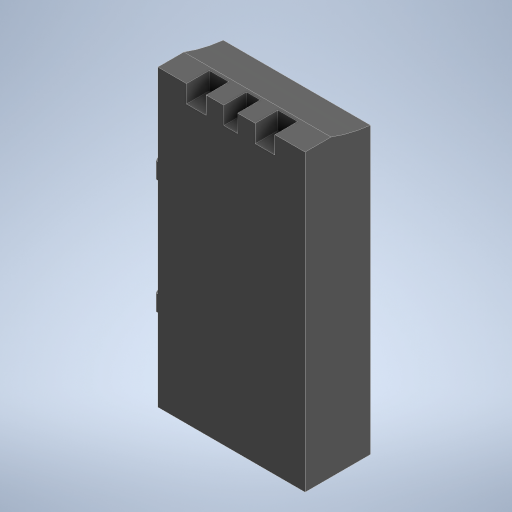
# Autodesk Inventor part: battery
Saved by Autodesk Inventor 2024.1 (Build 281209000, 209)
## iProperties
Created: 2025-03-04
Part Number: battery
Material: 一般
Document SubType Name: Modeling
Designer: hibik
Density: 1 g/cm^3
Appearance: 既定
Author: hibik
Autodesk Inventor part; units mm, degrees
ref_plane "YZ Plane" through (0, 0, 0) normal (1, 0, 0) x (0, 1, 0)
ref_plane "XZ Plane" through (0, 0, 0) normal (0, 1, 0) x (-1, 0, 0)
ref_plane "XY Plane" through (0, 0, 0) normal (0, 0, 1) x (1, 0, 0)
sketch "スケッチ1" plane through (0, 0, 0) normal (0, 1, 0) x (-1, 0, 0)
  line L0 (-22.5, -10) -> (22.5, -10)
  line L1 (22.5, -10) -> (22.5, 10)
  line L2 (22.5, 10) -> (-22.5, 10)
  line L3 (-22.5, 10) -> (-22.5, -10)
  line L4 (-22.5, -10) -> (22.5, 10) construction
  line L5 (22.5, -10) -> (-22.5, 10) construction
  point P0 (0, 0)
  dimension "d0" = 45
  dimension "d1" = 20
  constraints: 12 end point, 2 midpoint, 2 parallel, 1 horizontal, 1 perpendicular
  measures "d0" distance of L2.end L1.end
  measures "d1" distance of L1.end L0.end
extrude "押し出し1" add sketch "スケッチ1" along normal blind 90
sketch "スケッチ2" plane through (-22.5, 0, 10) normal (0, 0, 1) x (1, 0, 0)
  line L0 (0, 0) -> (0, 90) projected
  line L1 (0, 65) -> (-3, 65)
  line L2 (-3, 65) -> (-3, 60)
  line L3 (-3, 60) -> (0, 60)
  line L4 (0, 60) -> (0, 65)
  line L5 (-3, 67.5) -> (-5, 67.5)
  line L6 (-5, 67.5) -> (-5, 57.5)
  line L7 (-5, 57.5) -> (-3, 57.5)
  line L8 (-3, 57.5) -> (-3, 67.5)
  line L9 (0, 90) -> (45, 90) projected
  point P0 (22.5, 0)
  point P1 (-5, 62.5)
  point P2 (-3, 62.5)
  point P3 (-3, 60)
  point P4 (0, 60)
  point P5 (-3, 65)
  dimension "d14" = 5
  dimension "d15" = 10
  dimension "d16" = 2
  dimension "d17" = 3
  dimension "d18" = 25
  constraints: 16 end point, 4 parallel, 2 horizontal, 2 midpoint, 2 perpendicular, 1 collinear, 1 horizontal alignment, 1 point on line
  measures "d14" distance of L1.end L2.end
  measures "d15" distance of L5.end L6.end
  measures "d16" distance of L5.start L5.end
  measures "d17" distance of L1.start L1.end
  measures "d18" distance between parallel lines of L9 L1
ref_plane "作業平面1" through (0, 45, 0) normal (0, 1, 0) x (1, 0, 0)
extrude "押し出し2" add sketch "スケッチ2" against normal up to surface (20 mm away)
mirror "ミラー1" about plane through (0, 45, 0) normal (0, 1, 0) of "押し出し2"
sketch "スケッチ3" plane through (-27.5, 67.5, 10) normal (0, 1, 0) x (1, 0, 0)
  line L0 (4.5, 0) -> (-25.5, 51.9615) projected
  line L1 (2, 20) -> (0, 20) projected
  line L2 (0, 0) -> (0, 20) projected
  line L3 (2, 0) -> (0, 0) projected
  line L4 (2, 0) -> (2, 20) projected
  line L5 (5, 20) -> (2, 20) projected
  line L6 (2, 0) -> (2, 20) projected
  line L7 (5, 0) -> (2, 0) projected
  line L8 (5, 20) -> (5, 0) projected
  point P0 (27.5, 10)
  point P1 (4.5, 0)
  point P2 (0, 7.7942)
extrude "押し出し3" cut sketch "スケッチ3" against normal through all contours L7 L4 L0 | L4 L3 L2 L0
sketch "スケッチ4" plane through (22.5, 0, 10) normal (1, 0, 0) x (0, 0, -1)
  line L0 (6.75, 91.5264) -> (6.75, 84.8044) projected
  line L1 (6.75, 84.8044) -> (1.25, 88.8044) projected
  line L2 (1.25, 91.5264) -> (1.25, 88.8044) projected
  line L3 (20, 90) -> (0, 90) projected
  line L4 (6.95, 90) -> (6.95, 84.6044)
  line L5 (6.95, 84.6044) -> (0, 84.6044)
  line L6 (0, 0) -> (0, 90) projected
  line L7 (0, 90) -> (20, 90) projected
  arc A0 (7.95, 90) -> (20, 87.1044) centre (25.5674, 136.7934) ccw
  line L8 (20, 0) -> (20, 90) projected
  point P0 (10, 0)
  point P1 (7.95, 90)
  dimension "d26" = 0.2
  dimension "d27" = 0.2
  dimension "d28" = 50
  dimension "d29" = 1
  dimension "d32" = 2.5
  constraints: 4 end point, 4 point on line, 2 perpendicular, 2 point on circle, 1 centre point, 1 vertical
  measures "d26" distance from line of L0.end L5
  measures "d27" distance between parallel lines of L0 L4
  measures "d28" radius of A0
  measures "d29" distance from line of L4 A0.start
  measures "d32" distance from line of A0.end L5
extrude "押し出し4" cut sketch "スケッチ4" against normal through all
sketch "スケッチ5" plane through (22.5, 84.6044, 3.05) normal (0, 0, 1) x (1, 0, 0)
  line L0 (-36.25, 5.3956) -> (-36.25, 12.3956)
  line L1 (-30.25, 6.8956) -> (-30.25, 5.3956)
  line L2 (-24.85, 10.8956) -> (-24.85, 5.3956)
  line L3 (-20.65, 5.3956) -> (-20.65, 10.8956)
  line L4 (-24.85, 10.8956) -> (-24.85, 5.3956)
  line L5 (-15.25, 5.3956) -> (-15.25, 6.8956)
  line L6 (-9.25, 12.3956) -> (-9.25, 5.3956)
  line L7 (0, 0) -> (-45, 0)
  line L8 (-36.25, 5.3956) -> (-45, 5.3956)
  line L9 (-45, 5.3956) -> (-45, 0)
  line L10 (-45, 0) -> (-36.25, 0)
  line L11 (-36.25, 0) -> (-36.25, 5.3956)
  line L12 (-30.25, 5.3956) -> (-24.85, 5.3956)
  line L13 (-24.85, 5.3956) -> (-24.85, 0)
  line L14 (-24.85, 0) -> (-30.25, 0)
  line L15 (-30.25, 0) -> (-30.25, 5.3956)
  line L16 (-20.65, 5.3956) -> (-15.25, 5.3956)
  line L17 (-15.25, 5.3956) -> (-15.25, 0)
  line L18 (-15.25, 0) -> (-20.65, 0)
  line L19 (-20.65, 0) -> (-20.65, 5.3956)
  line L20 (-9.25, 5.3956) -> (0, 5.3956)
  line L21 (0, 5.3956) -> (0, 0)
  line L22 (0, 0) -> (-9.25, 0)
  line L23 (-9.25, 0) -> (-9.25, 5.3956)
  point P0 (-22.5, -84.6044)
  point P1 (-9.25, 0)
extrude "押し出し5" add sketch "スケッチ5" along normal up to surface (6.95 mm away)
equation "\"d27\" = d26"
